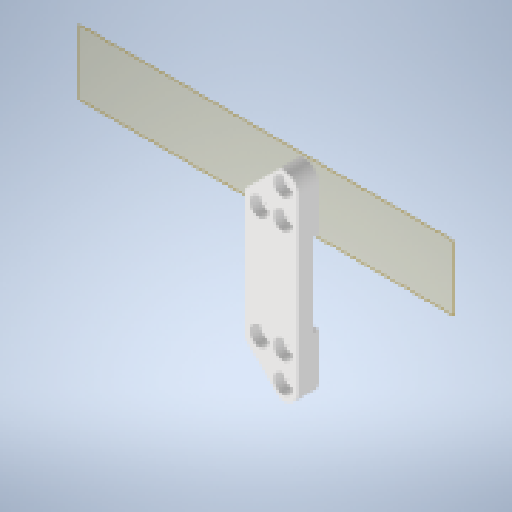
# Autodesk Inventor part: SideBrace
Saved by Autodesk Inventor 2023 (Build 270158000, 158)
## iProperties
Created: 2023-09-08
Part Number: SideBrace
Material: Generic
Document SubType Name: Modeling
Designer: Felix
Density: 1 g/cm^3
Appearance: Default
Mass: 6.93556 g
Surface Area: 38.2175 cm^2
Volume: 6.93556 cm^3
Author: Felix
Autodesk Inventor part; units mm, degrees
ref_plane "YZ Plane" through (0, 0, 0) normal (1, 0, 0) x (0, 1, 0)
ref_plane "XZ Plane" through (0, 0, 0) normal (0, 1, 0) x (-1, 0, 0)
ref_plane "XY Plane" through (0, 0, 0) normal (0, 0, 1) x (1, 0, 0)
ref_plane "Work Plane1" through (0, 0, 0) normal (0, 0, 1) x (1, 0, 0)
sketch "Sketch1" plane through (0, 0, 0) normal (0, 0, 1) x (1, 0, 0)
  line L0 (-32.75, 0) -> (32.75, 0) projected
  arc A0 (37.75, -5) -> (32.75, 0) centre (32.75, -5) ccw projected
  line L1 (37.75, -5) -> (37.75, -15) projected
  line L2 (-37.75, -20) -> (77.75, -20) construction
  line L3 (0.95, -48) -> (37.75, -48) construction
  arc A1 (32.75, -68) -> (37.75, -63) centre (32.75, -63) ccw projected
  line L4 (37.75, -63) -> (37.75, -48) projected
  line L5 (26.6, -68) -> (32.75, -68) projected
  line L6 (19.75, 0) -> (37.75, 0)
  line L7 (37.75, 0) -> (37.75, -68)
  line L8 (37.75, -68) -> (19.75, -68)
  line L9 (19.75, -68) -> (19.75, 0)
  point P0 (0, 0)
  point P1 (24.75, -5)
  point P2 (24.75, -63)
  dimension "d0" = 18
  dimension "d1" = 5
  dimension "d2" = 5
  dimension "d3" = 5
  constraints: 8 end point, 3 point on line, 2 horizontal alignment, 2 parallel, 1 horizontal, 1 perpendicular
  measures "d0" distance between parallel lines of L1 L9
  measures "d1" distance from line of L1 A0.centre
  measures "d2" distance from line of L9 point (24.75, -5)
  measures "d3" distance from line of point (24.75, -63) L9
extrude "Extrusion1" add sketch "Sketch1" along normal blind 7 contours L0 A0 L1 L7 L4 A1 L5 L8 L9
sketch "Sketch2" plane through (0, 0, 0) normal (0, 0, -1) x (-1, 0, 0)
  line L0 (37.75, -20) -> (-77.75, -20) construction
  line L1 (-0.95, -48) -> (-37.75, -48) projected
  line L2 (-19.75, 0) -> (-19.75, -68) projected
  line L3 (-37.75, -63) -> (-37.75, -5) projected
  line L4 (-19.75, -48) -> (-37.75, -48)
  line L5 (-37.75, -48) -> (-37.75, -20)
  line L6 (-37.75, -20) -> (-19.75, -20)
  line L7 (-19.75, -20) -> (-19.75, -48)
  point P0 (0, 0)
  point P1 (-19.75, -20)
  constraints: 8 end point, 4 point on line, 2 parallel, 1 horizontal, 1 perpendicular
extrude "Extrusion2" cut sketch "Sketch2" against normal blind 2
sketch "Sketch3" plane through (0, 0, 7) normal (0, 0, 1) x (1, 0, 0)
  line L0 (19.75, -68) -> (32.75, -68) projected
  arc A0 (32.75, -68) -> (37.75, -63) centre (32.75, -63) ccw projected
  line L1 (37.75, -63) -> (37.75, -5) projected
  arc A1 (37.75, -5) -> (32.75, 0) centre (32.75, -5) ccw projected
  line L2 (32.75, 0) -> (19.75, 0) projected
  line L3 (19.75, 0) -> (19.75, -68) projected
  line L4 (37.75, -34) -> (19.75, -34) construction
  line L5 (28.75, -34) -> (28.75, -68) construction
  line L6 (19.75, -68) -> (32.75, -68) projected
  line L7 (-37.75, -20) -> (77.75, -20) construction
  line L8 (0.95, -48) -> (37.75, -48) projected
  line L9 (77.75, -15) -> (37.75, -15) projected
  point P0 (0, 0)
  point P1 (32.75, -63)
  point P2 (32.75, -15)
  point P3 (32.75, -53)
  point P4 (24.75, -15)
  point P5 (24.75, -53)
  dimension "d15" = 5
  dimension "d16" = 5
  dimension "d22" = 5
  dimension "d23" = 5
  constraints: 4 end point, 4 symmetric about line, 3 midpoint, 1 coincident, 1 perpendicular, 1 point on line
  measures "d15" distance from line of L1 point (32.75, -5)
  measures "d16" distance from line of L1 point (32.75, -15)
  measures "d22" distance between parallel lines of L7 L9
  measures "d23" distance from line of L7 point (32.75, -15)
hole "Hole1" at (32.75, -5, 7) at (32.75, -63, 7) at (32.75, -15, 7) at (24.75, -15, 7) at (24.75, -53, 7) at (32.75, -53, 7) direction (0, 0, -1) diameter 3.4 depth 7 counterbore diameter 6.5 counterbore depth 3.4 clearance for "Socket Head Cap Screw DIN EN ISO 4762" size "M3" standard "DIN"
chamfer "Chamfer1" distance 12 angle 45 2 edges at (19.75, -68, 3.5) (19.75, 0, 3.5)
equation "\"d2\" = d1"
equation "\"d3\" = d1"
equation "\"d16\" = d15"
body "Solid1"
